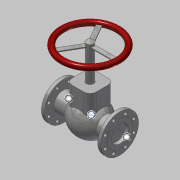
# Autodesk Inventor part: µGLOBE VALVE FLANGED DN100
Saved by Autodesk Inventor 2017 (Build 210142000, 142)
## iProperties
Category: Piping Part
Company: Demarec
Created: 2012-12-20
Part Number: µGLOBE VALVE FLANGED DN100
Material: S235
Document SubType Name: Modeling
Designer: Marc Crauwels
Density: 7.85 g/cm^3
Mass: 658107 g
Surface Area: 21375.3 cm^2
Volume: 83622.3 cm^3
Appearance: Steel
Catalog Web Link: http://www.pocketbrewery.com
Author: Marc Crauwels
Title: Carbon Steel Globe Valve PN16
Comments: iPart CS GlbVlvPN16
Autodesk Inventor part; units mm, degrees
ref_plane "YZ Plane" through (0, 0, 0) normal (1, 0, 0) x (0, 1, 0)
ref_plane "XZ Plane" through (0, 0, 0) normal (0, 1, 0) x (-1, 0, 0)
ref_plane "XY Plane" through (0, 0, 0) normal (0, 0, 1) x (1, 0, 0)
sketch "Sketch1" plane through (0, 0, 0) normal (1, 0, 0) x (0, 1, 0)
  line L0 (155, 50) -> (173, 50)
  line L1 (173, 50) -> (173, 110)
  line L2 (173, 110) -> (155, 110)
  line L3 (155, 110) -> (155, 50)
  line L4 (173, 50) -> (175, 50)
  line L5 (175, 50) -> (175, 76)
  line L6 (175, 76) -> (173, 76)
  line L7 (173, 76) -> (173, 50)
  line L8 (-175, 0) -> (175, 0) construction
  line L9 (175, 0) -> (155, 0) construction
  line L10 (0, 0) -> (0, 377) construction
  line L11 (-175, 0) -> (-155, 0) construction
  line L12 (0, 0) -> (-21.3333, 0)
  line L13 (-21.3333, 0) -> (-21.3333, 377)
  line L14 (-21.3333, 377) -> (0, 377)
  line L15 (0, 377) -> (0, 0)
  line L16 (-21.3333, 363.5) -> (-160, 363.5)
  line L17 (-160, 363.5) -> (-160, 358.5)
  line L18 (-160, 358.5) -> (-21.3333, 358.5)
  line L19 (-21.3333, 358.5) -> (-21.3333, 363.5)
  circle A0 centre (-160, 361) radius 16
  dimension "Lenght" = 350
  dimension "DN" = 100
  dimension "FlgDia" = 220
  dimension "FlgThck" = 20
  dimension "GsktFace" = 152
  dimension "Height" = 377
  dimension "d48" = 21.3333
  dimension "d49" = 32
  dimension "d50" = 5
  dimension "d51" = 160
  dimension "Face" = 2
  constraints: 40 end point, 8 parallel, 7 point on line, 5 perpendicular, 4 horizontal, 2 coincident, 2 collinear, 2 midpoint, 1 centre point, 1 tangent
  measures "Lenght" distance of L8.start L8.end
  measures "DN" diameter of L0 L8
  measures "FlgDia" diameter of L2 L8
  measures "FlgThck" distance between parallel lines of L3 L5
  measures "GsktFace" diameter of L5.end L8
  measures "Height" distance of L10.start L10.end
  measures "d48" distance of L13.end L14.end
  measures "d49" diameter of A0
  measures "d50" distance of L16.end L17.end
  measures "d51" distance from line of A0.centre L10
  measures "Face" distance of L5.end L6.end
revolve "Revolution1" add sketch "Sketch1" angle 360 about axis through (0, -175, 0) along (0, 1, 0) contours L3 L2 L1 L0 | L1 L6 L5 L4
sketch "Sketch5" plane through (0, 175, 0) normal (0, 1, 0) x (1, 0, 0)
  line L0 (0, 0) -> (-34.4415, 83.1492)
  line L1 (0, 0) -> (0, 336) construction
  circle A0 centre (-34.4415, 83.1492) radius 9
  point P0 (0, 0)
  dimension "d16" = 90
  dimension "d17" = 22.5
  dimension "d18" = 18
  constraints: 4 end point, 2 coincident, 1 centre point, 1 vertical
  measures "d16" distance of L0.start L0.end
  measures "d17" angle of L1 L0
  measures "d18" diameter of A0
extrude "Extrusion2" cut sketch "Sketch5" against normal through all
pattern_circular "Circular Pattern1" count 8 over 360 about axis through (0, 174, 0) along (0, 1, 0) of "Extrusion2"
sketch "Sketch14" plane through (0, 155, 0) normal (0, -1, 0) x (-1, 0, 0)
  circle A0 centre (0, 0) radius 50 projected
  circle A1 centre (0, 0) radius 56
  dimension "d54" = 6
  constraints: 1 centre point
  measures "d54" radial gap between concentric circles of A1 A0
pattern_circular "Circular Pattern2" count 2 over 360 about axis through (-10, 0, 0) along (1, 0, 0) of "Revolution1", "Extrusion2", "Circular Pattern1"
extrude "Extrusion5" add sketch "Sketch14" along normal up to surface (310 mm away) contours A0 | A1
sketch "Sketch15" plane through (0, 0, 0) normal (0, 0, 1) x (1, 0, 0)
  line L0 (70, -70) -> (-70, -70)
  line L1 (-70, -70) -> (-70, 70)
  line L2 (-70, 70) -> (70, 70)
  line L3 (70, 70) -> (70, -70)
  line L4 (-70, -70) -> (70, 70) construction
  point P0 (0, 0)
  point P1 (0, 0)
  dimension "d57" = 140
  dimension "d59" = 140
  constraints: 10 end point, 2 parallel, 1 coincident, 1 horizontal, 1 midpoint, 1 perpendicular
  measures "d57" distance of L2.end L0.start
  measures "d59" distance of L0.start L0.end
extrude "Extrusion4" add sketch "Sketch15" along normal blind 176
sketch "Sketch17" plane through (-70, 0, 0) normal (-1, 0, 0) x (0, 0, 1)
  line L0 (176, 70) -> (176, -70) projected
  circle A0 centre (176, 0) radius 70
  point P0 (0, 0)
  constraints: 1 midpoint, 1 vertical alignment, 2 other
extrude "Extrusion7" [suppressed]
revolve "Revolution3" add sketch "Sketch1" angle 360 about axis through (0, 0, 0) along (0, 0, 1) contours L12 L13 L14 L15 | L18 A0 L16 L13 | A0 L16 L17 L18 | L18 L17 L16 A0
fillet "Fillet1" radius 35 4 edges at (70, -70, 88) (-70, -70, 88) (70, 70, 88) (-70, 70, 88)
sketch "Sketch16" plane through (0, 0, 363.5) normal (0, 0, 1) x (1, 0, 0)
  line L0 (0, 0) -> (0, 112.0641) construction
  line L1 (0, 0) -> (89.1399, 51.465) construction
  line L2 (0, 0) -> (-84.4387, 48.7507) construction
  line L3 (-117.9849, 82.8988) -> (-8.3802, 19.6185)
  line L4 (117.9849, 82.8988) -> (8.3802, 19.6185)
  circle A0 centre (0, 0) radius 21.3333 projected
  circle A1 centre (0, 0) radius 144.1965 projected
  arc A2 (8.3802, 19.6185) -> (-8.3802, 19.6185) centre (0, 0) ccw
  arc A3 (117.9849, 82.8988) -> (-117.9849, 82.8988) centre (0, 0) ccw
  dimension "d61" = 120
  dimension "d62" = 60
  dimension "d63" = 12.8
  dimension "d64" = 12.8
  constraints: 10 end point, 8 point on circle, 2 centre point, 2 coincident, 2 concentric, 2 parallel, 1 vertical
  measures "d61" angle of L1 L2
  measures "d62" angle of L0 L1
  measures "d63" distance between parallel lines of L3 L2
  measures "d64" distance between parallel lines of L1 L4
extrude "Extrusion6" cut sketch "Sketch16" against normal blind 5 contours A1 L4 A0 L3 picked at (-78.0915, 66.0545)
pattern_circular "Circular Pattern3" count 3 over 360 about axis through (0, 0, 370.25) along (0, 0, 1) of "Extrusion6"
sketch "Sketch19" plane through (0, 0, 0) normal (1, 0, 0) x (0, 1, 0)
  line L0 (155, -56) -> (-155, -56)
  line L1 (91.2725, -56) -> (-91.2725, -56)
  arc A0 (-91.2725, -56) -> (91.2725, -56) centre (0, 16.6667) ccw
  line L2 (183.9666, 0) -> (-194.0334, 0)
  line L3 (0, 16.6667) -> (0, 0) construction
  line L4 (0, 0) -> (0, -100) construction
  line L5 (0, -135.593) -> (0, 9.0736)
  line L6 (0, -276.6667) -> (0, 120) projected
  line L7 (-555.8, 0) -> (555.8, 0) projected
  line L8 (155, -56) -> (-155, -56) projected
  point P0 (0, -56)
  dimension "d75" = 116.6667
  dimension "d77" = 100
  constraints: 12 end point, 3 collinear, 3 point on circle, 2 midpoint, 2 point on line, 1 centre point, 1 horizontal, 1 perpendicular
  measures "d75" radius of A0
  measures "d77" distance of L3.end L4.end
revolve "Revolution4" add sketch "Sketch19" angle 360 about axis through (0, 183.9666, 0) along (0, -1, 0)
equation "\"d51\" = 0.5 * WhlDia"
equation "\"d16\" = 0.5 * KDia"
equation "\"WhlDia\" = 320"
equation "\"KDia\" = 180"
body "Solid1"
